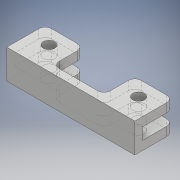
# Autodesk Inventor part: Suporte Carretel
Saved by Autodesk Inventor 2017 (Build 210142000, 142)
## iProperties
Created: 2020-10-18
Part Number: Suporte Carretel
Material: Generic
Document SubType Name: Modeling
Designer: ale
Density: 1 g/cm^3
Appearance: Default
Author: ale
Autodesk Inventor part; units mm, degrees
ref_plane "YZ Plane" through (0, 0, 0) normal (1, 0, 0) x (0, 1, 0)
ref_plane "XZ Plane" through (0, 0, 0) normal (0, 1, 0) x (-1, 0, 0)
ref_plane "XY Plane" through (0, 0, 0) normal (0, 0, 1) x (1, 0, 0)
sketch "Sketch1" plane through (0, 0, 0) normal (0, 0, 1) x (1, 0, 0)
  line L0 (10, 15) -> (-10, 15)
  line L1 (-15, 10) -> (-15, -15)
  line L2 (-15, -15) -> (15, -15)
  line L3 (15, -4) -> (15, 10)
  line L4 (15, 15) -> (-15, -15) construction
  line L5 (-15, 15) -> (15, -15) construction
  line L6 (15, -15) -> (55, -15)
  line L7 (85, -15) -> (85, -9)
  line L8 (-15, -9) -> (-15, -15)
  line L9 (85, -15) -> (55, -15)
  line L10 (55, -4) -> (55, 10)
  line L11 (60, 15) -> (80, 15)
  line L12 (85, 10) -> (85, -15)
  line L13 (50, -9) -> (20, -9)
  arc A0 (-10, 15) -> (-15, 10) centre (-10, 10) ccw
  arc A1 (15, 10) -> (10, 15) centre (10, 10) ccw
  arc A2 (15, -4) -> (20, -9) centre (20, -4) ccw
  arc A3 (50, -9) -> (55, -4) centre (50, -4) ccw
  arc A4 (60, 15) -> (55, 10) centre (60, 10) ccw
  arc A5 (85, 10) -> (80, 15) centre (80, 10) ccw
  point P0 (0, 0)
  point P1 (55, 15)
  point P2 (85, 15)
  dimension "d0" = 30
  dimension "d1" = 30
  dimension "d2" = 100
  dimension "d3" = 6
  dimension "d4" = 30
  dimension "d5" = 30
  dimension "d6" = 5
  constraints: 28 end point, 12 point on circle, 12 tangent, 8 point on line, 6 centre point, 6 parallel, 5 equal radius, 3 horizontal, 3 perpendicular, 2 midpoint
  measures "d0" distance of L2.end L1.end
  measures "d1" distance of L1.end L5.start
  measures "d2" distance of L8.start L7.end
  measures "d3" distance of L7.end L7.start
  measures "d4" distance of point (55, 15) point (85, 15)
  measures "d5" distance of L6.end point (55, 15)
  measures "d6" radius of A0
extrude "Extrusion1" add sketch "Sketch1" along normal blind 7
ref_plane "Work Plane1" through (0, 0, 11.5) normal (0, 0, 1) x (1, 0, 0)
mirror "Mirror1" about plane through (0, 0, 11.5) normal (0, 0, 1)
sketch "Sketch3" plane through (0, 0, 7) normal (0, 0, 1) x (1, 0, 0)
  line L0 (-15, -15) -> (85, -15)
  line L1 (85, -15) -> (85, -9)
  line L2 (85, -9) -> (-15, -9)
  line L3 (-15, -9) -> (-15, -15)
  point P0 (0, 0)
  dimension "d14" = 100
  dimension "d15" = 6
  constraints: 8 end point, 2 parallel, 1 horizontal, 1 perpendicular
  measures "d14" distance of L2.end L1.end
  measures "d15" distance of L1.end L0.end
extrude "Extrusion3" add sketch "Sketch3" along normal blind 9
sketch "Sketch4" plane through (0, 0, 0) normal (0, 0, -1) x (-1, 0, 0)
  line L0 (-60, 15) -> (-80, 15) projected
  line L1 (-55, -4) -> (-55, 10) projected
  line L2 (-85, -15) -> (15, -15) projected
  line L3 (-35, -15) -> (-35, -9)
  line L4 (-20, -9) -> (-50, -9) projected
  point P0 (0, 0)
  point P1 (-70, 3)
  point P2 (0, 3)
  dimension "d18" = 12
  dimension "d19" = 15
  constraints: 2 end point, 2 midpoint, 1 symmetric about line
  measures "d18" distance from line of point (-70, 3) L0
  measures "d19" distance from line of L1 point (-70, 3)
hole "Hole1" at (70, 3, 0) at (0, 3, 0) direction (0, 0, 1) diameter 9 end through all
body "Solid1"
